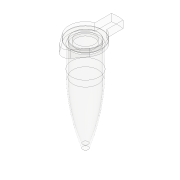
# Autodesk Inventor part: Vial
Saved by Autodesk Inventor 2017 (Build 210142000, 142)
## iProperties
Created: 2016-08-01
Part Number: Vial
Material: Glass
Document SubType Name: Modeling
Designer: ge937963
Density: 2.18 g/cm^3
Appearance: Transparent - Clear
Author: ge937963
Autodesk Inventor part; units mm, degrees
ref_plane "YZ Plane" through (0, 0, 0) normal (1, 0, 0) x (0, 1, 0)
ref_plane "XZ Plane" through (0, 0, 0) normal (0, 1, 0) x (-1, 0, 0)
ref_plane "XY Plane" through (0, 0, 0) normal (0, 0, 1) x (1, 0, 0)
sketch "Sketch1" plane through (0, 0, 0) normal (0, 0, 1) x (1, 0, 0)
  line L0 (3, 15.24) -> (3, 20)
  line L1 (3, 20) -> (2.7, 20)
  line L2 (2.7, 20) -> (2.7, 13.7288)
  line L3 (0, 0.6837) -> (0, 0)
  arc A0 (0, 0) -> (0.5935, 0.4276) centre (0, 0.6256) ccw
  arc A1 (0.5935, 0.4276) -> (3, 15.24) centre (-43.7889, 15.24) ccw
  line L4 (0, 0) -> (-1.9294, 0)
  arc A2 (0, 0.6837) -> (0.5584, 1.3498) centre (-0.6188, 1.7696) ccw
  arc A3 (0.5584, 1.3498) -> (2.7, 13.7288) centre (-34.1481, 13.7288) ccw
  line L5 (-6.5051, 6.35) -> (10.1936, 6.35)
  line L6 (2.1819, 6.35) -> (2.1819, 2.9816)
  dimension "d0" = 3
  dimension "d1" = 15.24
  dimension "d2" = 20
  dimension "d3" = 2.7
  dimension "d7" = 6.35
  dimension "d8" = 2.1819
  constraints: 14 end point, 8 point on circle, 5 tangent, 4 centre point, 3 horizontal, 2 vertical, 1 parallel, 1 perpendicular, 1 point on line
  measures "d0" distance between parallel lines of L0 L3
  measures "d1" vertical distance of L0.start L3.end
  measures "d2" distance from line of L3.end L1
  measures "d3" distance from line of L3.start L2
  measures "d7" distance from line of L5 L3.end
  measures "d8" distance between parallel lines of L3 L6
revolve "Revolution1" add sketch "Sketch1" angle 360 about axis through (0, 0.6837, 0) along (0, -1, 0)
sketch "Sketch2" plane through (0, 20, 0) normal (0, 1, 0) x (1, 0, 0)
  circle A0 centre (0, 0) radius 3.556
  circle A1 centre (0, 0) radius 2.7
  dimension "d9" = 7.112
  constraints: 2 centre point, 2 coincident
  measures "d9" diameter of A0
extrude "Extrusion1" add sketch "Sketch2" along normal blind 0.762
sketch "Sketch3" plane through (0, 0, 0) normal (1, 0, 0) x (0, 1, 0)
  line L0 (21.5893, 0) -> (20.8527, 0)
  line L1 (20.8527, 0) -> (20.8527, -6.985)
  line L2 (20.8527, -6.985) -> (21.5893, -6.985)
  line L3 (21.5893, -6.985) -> (21.5893, 0)
  line L4 (20.762, -3.556) -> (20.762, 3.556) projected
  line L5 (20, 3.556) -> (20, -3.556) projected
  line L6 (20.8527, -2.6155) -> (20, -2.6155)
  line L7 (20, -2.6155) -> (20, -1.9879)
  line L8 (20, -1.9879) -> (20.8527, -1.9879)
  line L9 (20.8527, -1.9879) -> (20.8527, -2.6155)
  point P0 (0, 0)
  point P1 (20.762, 0)
  dimension "d12" = 6.985
  dimension "d13" = 0.7366
  constraints: 16 end point, 4 parallel, 2 horizontal, 2 perpendicular, 2 point on line, 1 horizontal alignment, 1 midpoint
  measures "d12" distance of L2.end L0.start
  measures "d13" distance of L0.start L0.end
revolve "Revolution2" add sketch "Sketch3" angle 360 about axis through (0, 21.5893, 0) along (0, -1, 0)
sketch "Sketch4" plane through (0, 21.5893, 0) normal (0, 1, 0) x (1, 0, 0)
  line L0 (-1.1941, -4.4189) -> (-2.8822, -2.0828)
  circle A0 centre (0, 0) radius 3.556 projected
  line L1 (2.8822, -2.0828) -> (1.1941, -4.4189)
  line L2 (1.27, 3.3215) -> (1.27, 6.8686)
  circle A1 centre (0, 0) radius 6.985 projected
  line L3 (-1.27, 3.3215) -> (-1.27, 6.8686)
  line L4 (-1.27, 6.8686) -> (1.27, 6.8686)
  circle A2 centre (0, 0) radius 3.556 projected
  arc A3 (-1.1941, -4.4189) -> (1.1941, -4.4189) centre (0, -3.556) ccw
  line L5 (0, -5.0292) -> (-1.1247, -5.0292)
  point P0 (0, 6.8686)
  dimension "d15" = 2.54
  dimension "d16" = 5.0292
  constraints: 12 end point, 10 point on circle, 4 tangent, 3 vertical alignment, 1 centre point, 1 horizontal, 1 midpoint, 1 parallel, 1 perpendicular, 1 vertical, 1 other
  measures "d15" distance of L3.end L2.end
  measures "d16" distance from line of point (0, 0) L5
extrude "Extrusion2" cut sketch "Sketch4" against normal blind 25.4 contours A3 L1 A0 L2 A1 L3 L0
sketch "Sketch5" plane through (0, 20.8527, 3.556) normal (0, -1, 0) x (1, 0, 0)
  circle A0 centre (0, -3.556) radius 3.556 projected
  circle A1 centre (0, -3.556) radius 2.6155 projected
  line L0 (1.27, -10.4246) -> (1.27, -6.8775) projected
  arc A2 (1.27, -6.8775) -> (2.8822, -1.4732) centre (0, -3.556) ccw projected
  line L1 (2.8822, -1.4732) -> (1.1941, 0.8629) projected
  arc A3 (1.1941, 0.8629) -> (-1.1941, 0.8629) centre (0, 0) ccw projected
  line L2 (-1.1941, 0.8629) -> (-2.8822, -1.4732) projected
  arc A4 (-2.8822, -1.4732) -> (-1.27, -6.8775) centre (0, -3.556) ccw projected
  line L3 (-1.27, -6.8775) -> (-1.27, -10.4246) projected
  arc A5 (-1.27, -10.4246) -> (1.27, -10.4246) centre (0, -3.556) ccw projected
extrude "Extrusion3" add sketch "Sketch5" along normal up to surface (0.8527 mm away) contours A0 L2 A3 L1 | L0 A5 L3 A0
body "Solid1"
